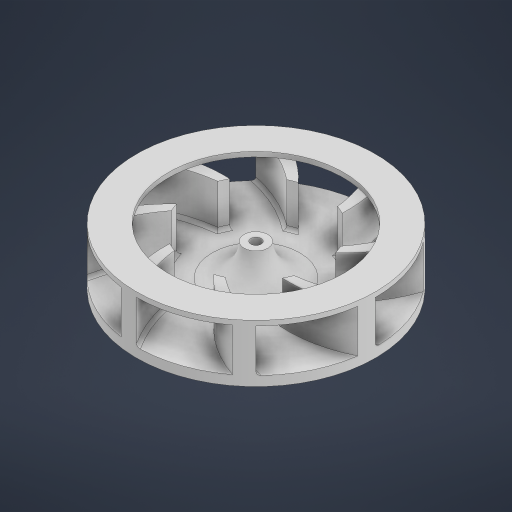
# Autodesk Inventor part: Fan4
Saved by Autodesk Inventor 2023 (Build 270158000, 158)
## iProperties
Created: 2022-10-05
Part Number: Fan4
Material: 一般
Document SubType Name: Modeling
Designer: neko2
Density: 1 g/cm^3
Appearance: 既定
Author: neko2
Autodesk Inventor part; units mm, degrees
ref_plane "YZ Plane" through (0, 0, 0) normal (1, 0, 0) x (0, 1, 0)
ref_plane "XZ Plane" through (0, 0, 0) normal (0, 1, 0) x (-1, 0, 0)
ref_plane "XY Plane" through (0, 0, 0) normal (0, 0, 1) x (1, 0, 0)
sketch "スケッチ1" plane through (0, 0, 0) normal (0, 1, 0) x (-1, 0, 0)
  circle A0 centre (0, 0) radius 7.5
  dimension "d0" = 15
  constraints: 1 centre point, 1 coincident
  measures "d0" diameter of A0
extrude "押し出し1" add sketch "スケッチ1" along normal blind 0.6
sketch "スケッチ2" plane through (0, 0.6, 0) normal (0, 1, 0) x (1, 0, 0)
  circle A0 centre (0, 0) radius 7.5 projected
  circle A1 centre (0, 0) radius 4
  arc A2 (-1.3681, -3.7588) -> (0, -7.5) centre (7.559, -2.6151) ccw
  arc A3 (-1.8779, -3.5318) -> (-1.0438, -7.427) centre (6.1155, -3.8571) ccw
  line L0 (0, 0) -> (-1.3681, -3.7588)
  line L1 (-1.8779, -3.5318) -> (0, 0)
  line L2 (0, -7.5) -> (0, 0)
  line L3 (0, 0) -> (-1.0438, -7.427)
  dimension "d27" = 8
  dimension "d30" = 9
  dimension "d52" = 8
  dimension "d53" = 8
  dimension "d55" = 8
  dimension "d56" = 20
  constraints: 8 end point, 8 point on circle, 3 centre point, 1 coincident, 1 vertical, 1 vertical alignment
  measures "d27" diameter of A1
  measures "d30" radius of A2
  measures "d52" radius of A3
  measures "d53" angle of L0 L1
  measures "d55" angle of L2 L3
  measures "d56" angle of L2 L0
extrude "押し出し2" add sketch "スケッチ2" along normal blind 2.7 contours L3 A2 A0 | A3 A1 A2 L3
fillet "フィレット2" radius 0.2 2 edges at (-0.8936, 0.6, 5.706) (-1.6269, 0.6, 3.6542)
pattern_circular "円形状パターン3" count 8 over 360 about axis through (0, -10, 0) along (0, 1, 0)
sketch "スケッチ6" plane through (-4.456, 3.3, -1.3534) normal (0, 1, 0) x (0.7460152, 0, 0.665929)
  circle A0 centre (4.2256, 1.9577) radius 5.5
  circle A1 centre (4.2256, 1.9577) radius 7.5 projected
  circle A2 centre (4.2256, 1.9577) radius 7.5
  dimension "d38" = 2
  constraints: 2 centre point, 2 coincident, 1 concentric
  measures "d38" radial gap between concentric circles of A1 A0
extrude "押し出し6" add sketch "スケッチ6" along normal blind 0.3
sketch "スケッチ9" plane through (0, 0.6, 0) normal (0, 1, 0) x (1, 0, 0)
  circle A0 centre (0, 0) radius 0.75
  dimension "d44" = 1.5
  constraints: 1 centre point, 1 coincident
  measures "d44" diameter of A0
extrude "押し出し8" add sketch "スケッチ9" along normal blind 2
fillet "フィレット3" radius 2 1 edges at (-0.75, 0.6, 0)
sketch "スケッチ10" plane through (0, 2.6, 0) normal (0, 1, 0) x (1, 0, 0)
  circle A0 centre (0, 0) radius 0.325
  dimension "d48" = 0.65
  constraints: 1 centre point, 1 coincident
  measures "d48" diameter of A0
extrude "押し出し9" cut sketch "スケッチ10" against normal through all
